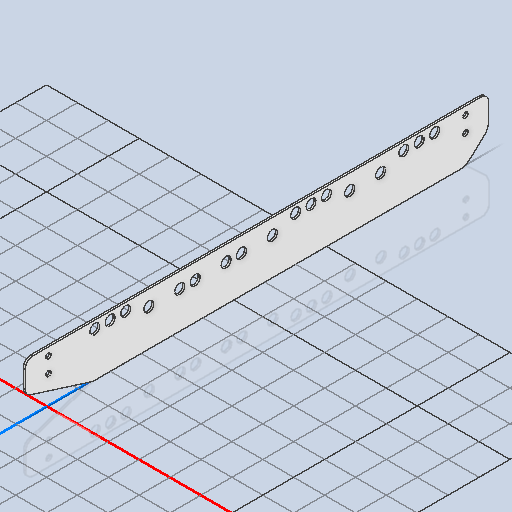
# Autodesk Inventor part: Skirt
Saved by Autodesk Inventor 2026 (Build 300175000, 175)
## iProperties
Created: 2025-04-07
Part Number: Skirt
Material: Acetal Resin, White
Document SubType Name: Modeling
Designer: avere
Density: 1.425 g/cm^3
Appearance: Smooth - White
Author: avere
Autodesk Inventor part; units mm, degrees
ref_plane "YZ Plane" through (0, 0, 0) normal (1, 0, 0) x (0, 1, 0)
ref_plane "XZ Plane" through (0, 0, 0) normal (0, 1, 0) x (-1, 0, 0)
ref_plane "XY Plane" through (0, 0, 0) normal (0, 0, 1) x (1, 0, 0)
sketch "main" plane through (0, 0, 0) normal (0, 0, 1) x (1, 0, 0)
  circle A0 centre (10.1168, 23.8511) radius 4.064
  circle A1 centre (10.1168, 11.1511) radius 4.064
  circle A2 centre (10.1168, -14.2489) radius 4.064
  circle A3 centre (16.4668, -33.2989) radius 4.0005
  circle A4 centre (16.4668, -58.6989) radius 4.0005
  circle A5 centre (10.1168, -77.7489) radius 4.064
  circle A6 centre (3.7668, 169.9011) radius 2.1844
  circle A7 centre (16.4668, 169.9011) radius 2.1844
  circle A8 centre (10.1168, -103.1489) radius 4.064
  circle A9 centre (16.4668, -122.1989) radius 4.0005
  circle A10 centre (3.7668, -172.9989) radius 2.1844
  circle A11 centre (16.4668, -172.9989) radius 2.1844
  line L0 (-20.0457, 131.4398) -> (-20.0457, -168.0589)
  line L1 (22.8168, -185.6989) -> (22.8168, 182.6011)
  line L2 (-16.7075, -176.6406) -> (-6.3583, -187.9307)
  line L3 (3.0036, -192.0489) -> (16.4668, -192.0489)
  arc A12 (-20.0457, -168.0589) -> (-16.7075, -176.6406) centre (-7.3457, -168.0589) ccw
  arc A13 (-6.3583, -187.9307) -> (3.0036, -192.0489) centre (3.0036, -179.3489) ccw
  circle A14 centre (16.4668, -147.5989) radius 4.0005
  arc A15 (16.4668, -192.0489) -> (22.8168, -185.6989) centre (16.4668, -185.6989) ccw
  line L4 (16.4668, 188.9511) -> (2.0773, 188.9511)
  line L5 (-3.9805, 184.505) -> (-19.4614, 135.2476)
  arc A16 (-19.4614, 135.2476) -> (-20.0457, 131.4398) centre (-7.3457, 131.4398) ccw
  circle A17 centre (10.1168, 49.2511) radius 4.064
  circle A18 centre (10.1168, 61.9511) radius 4.064
  circle A19 centre (10.1168, 87.3511) radius 4.064
  circle A20 centre (16.4668, 106.4011) radius 4.0005
  circle A21 centre (16.4668, 131.8011) radius 4.0005
  arc A22 (22.8168, 182.6011) -> (16.4668, 188.9511) centre (16.4668, 182.6011) ccw
  arc A23 (2.0773, 188.9511) -> (-3.9805, 184.505) centre (2.0773, 182.6011) ccw
  circle A24 centre (16.4668, 119.1011) radius 4.0005
  circle A25 centre (16.4668, -45.9989) radius 4.0005
  circle A26 centre (16.4668, -134.8989) radius 4.0005
  point P0 (5.8318, -6.3003)
  dimension "d16" = 12.7
  dimension "d17" = 6.35
  dimension "d18" = 6.35
  dimension "d19" = 8.001
  dimension "d20" = 25.4
  dimension "d21" = 165.1
  dimension "d22" = 254
  dimension "d23" = 8.128
  dimension "d24" = 25.4
  dimension "d25" = 38.1
  dimension "d26" = 25.4
  measures "d16" radius of A16
  measures "d17" radius of A23
  measures "d18" radius of A15
  measures "d19" diameter of A21
  measures "d20" distance of A21.centre A20.centre
  measures "d21" distance of A20.centre A4.centre
  measures "d22" distance of A20.centre A14.centre
  measures "d23" diameter of A19
  measures "d24" distance of A19.centre A18.centre
  measures "d25" distance of A18.centre A0.centre
  measures "d26" distance of A5.centre A8.centre
sketch "Sketch1" plane through (0, 0, 0) normal (1, 0, 0) x (0, 1, 0)
  circle A0 centre (6.35, -146.05) radius 4.064
  circle A1 centre (6.35, -158.75) radius 4.064
  circle A2 centre (6.35, -184.15) radius 4.064
  circle A3 centre (12.7, -203.2) radius 4.0005
  circle A4 centre (12.7, -228.6) radius 4.0005
  circle A5 centre (6.35, -247.65) radius 4.064
  circle A6 centre (0, 0) radius 2.1844
  circle A7 centre (12.7, 0) radius 2.1844
  circle A8 centre (6.35, -273.05) radius 4.064
  circle A9 centre (12.7, -292.1) radius 4.0005
  circle A10 centre (0, -342.9) radius 2.1844
  circle A11 centre (12.7, -342.9) radius 2.1844
  line L0 (-23.8125, -38.4612) -> (-23.8125, -337.9599)
  line L1 (19.05, -355.6) -> (19.05, 12.7)
  line L2 (-20.4744, -346.5416) -> (-10.1251, -357.8317)
  line L3 (-0.7632, -361.95) -> (12.7, -361.95)
  arc A12 (-23.8125, -337.9599) -> (-20.4744, -346.5416) centre (-11.1125, -337.9599) ccw
  arc A13 (-10.1251, -357.8317) -> (-0.7632, -361.95) centre (-0.7632, -349.25) ccw
  circle A14 centre (12.7, -317.5) radius 4.0005
  arc A15 (12.7, -361.95) -> (19.05, -355.6) centre (12.7, -355.6) ccw
  line L4 (12.7, 19.05) -> (-1.6895, 19.05)
  line L5 (-7.7473, 14.6039) -> (-23.2282, -34.6534)
  arc A16 (-23.2282, -34.6534) -> (-23.8125, -38.4612) centre (-11.1125, -38.4612) ccw
  circle A17 centre (6.35, -120.65) radius 4.064
  circle A18 centre (6.35, -107.95) radius 4.064
  circle A19 centre (6.35, -82.55) radius 4.064
  circle A20 centre (12.7, -63.5) radius 4.0005
  circle A21 centre (12.7, -38.1) radius 4.0005
  arc A22 (19.05, 12.7) -> (12.7, 19.05) centre (12.7, 12.7) ccw
  arc A23 (-1.6895, 19.05) -> (-7.7473, 14.6039) centre (-1.6895, 12.7) ccw
  circle A24 centre (12.7, -50.8) radius 4.0005
  circle A25 centre (12.7, -215.9) radius 4.0005
  circle A26 centre (12.7, -304.8) radius 4.0005
  constraints: 1 other
extrude "Extrusion1" add sketch "Sketch1" along normal blind 1.5875
body "Solid1"
